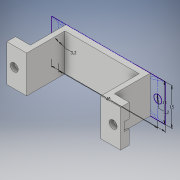
# Autodesk Inventor part: krepl_akum_line_racer
Saved by Autodesk Inventor 2019 (Build 230136000, 136)
## iProperties
Created: 2019-06-10
Part Number: krepl_akum_line_racer
Material: Типовые
Document SubType Name: Modeling
Designer: Администратор
Density: 1 g/cm^3
Appearance: По умолчанию
Author: Администратор
Autodesk Inventor part; units mm, degrees
ref_plane "YZ Plane" through (0, 0, 0) normal (1, 0, 0) x (0, 1, 0)
ref_plane "XZ Plane" through (0, 0, 0) normal (0, 1, 0) x (-1, 0, 0)
ref_plane "XY Plane" through (0, 0, 0) normal (0, 0, 1) x (1, 0, 0)
sketch "Эскиз1" plane through (0, 0, 0) normal (0, 0, 1) x (1, 0, 0)
  line L0 (-23, 7.5) -> (23, 7.5)
  line L1 (23, 7.5) -> (23, -7.5)
  line L2 (23, -7.5) -> (-23, -7.5)
  line L3 (-23, -7.5) -> (-23, 7.5)
  line L4 (-23, 7.5) -> (23, -7.5) construction
  line L5 (23, 7.5) -> (-23, -7.5) construction
  line L6 (-20, 7.5) -> (20, 7.5) construction
  line L7 (20, 7.5) -> (20, -7.5) construction
  line L8 (20, -7.5) -> (-20, -7.5) construction
  line L9 (-20, -7.5) -> (-20, 7.5) construction
  line L10 (-20, 7.5) -> (20, -7.5) construction
  line L11 (20, 7.5) -> (-20, -7.5) construction
  circle A0 centre (-20, 0) radius 1.6
  circle A1 centre (20, 0) radius 1.6
  point P0 (0, 0)
  dimension "d0" = 46
  dimension "d1" = 15
  dimension "d2" = 40
  dimension "d3" = 15
  dimension "d4" = 3.2
  dimension "d5" = 3.2
  constraints: 24 end point, 6 midpoint, 4 parallel, 2 centre point, 2 horizontal, 2 perpendicular
  measures "d0" distance of L1.end L2.end
  measures "d1" distance of L0.end L1.end
  measures "d2" distance of L7.end L8.end
  measures "d3" distance of L6.end L7.end
  measures "d4" diameter of A0
  measures "d5" diameter of A1
extrude "Выдавливание1" add sketch "Эскиз1" along normal blind 18
sketch "Эскиз2" plane through (0, 0, 18) normal (0, 0, 1) x (1, 0, 0)
  line L0 (-15, 7.5) -> (15, 7.5)
  line L1 (15, 7.5) -> (15, -7.5)
  line L2 (15, -7.5) -> (-15, -7.5)
  line L3 (-15, -7.5) -> (-15, 7.5)
  line L4 (-15, 7.5) -> (15, -7.5) construction
  line L5 (15, 7.5) -> (-15, -7.5) construction
  point P0 (0, 0)
  dimension "d8" = 30
  dimension "d9" = 15
  constraints: 12 end point, 2 midpoint, 2 parallel, 1 horizontal, 1 perpendicular
  measures "d8" distance of L1.end L2.end
  measures "d9" distance of L0.end L1.end
extrude "Выдавливание2" cut sketch "Эскиз2" against normal blind 15.5
sketch "Эскиз3" plane through (0, 0, 0) normal (0, 0, -1) x (-1, 0, 0)
  line L0 (-15, 7.5) -> (-15, -7.5) projected
  line L1 (15, -7.5) -> (15, 7.5) projected
  circle A0 centre (-20, 0) radius 1.6 projected
  circle A1 centre (20, 0) radius 1.6 projected
  line L2 (23, 7.5) -> (-23, 7.5) projected
  line L3 (-23, 7.5) -> (-23, -7.5) projected
  line L4 (-23, -7.5) -> (23, -7.5) projected
  line L5 (23, -7.5) -> (23, 7.5) projected
  line L6 (23, 7.5) -> (23, -7.5) projected
  line L7 (23, 7.5) -> (-23, 7.5) projected
  line L8 (23, -7.5) -> (17, -7.5)
  line L9 (17, -7.5) -> (17, 7.5)
  line L10 (17, 7.5) -> (23, 7.5)
  line L11 (23, 7.5) -> (23, -7.5)
  line L12 (-23, -7.5) -> (-23, 7.5) projected
  line L13 (-23, -7.5) -> (-17, -7.5)
  line L14 (-17, -7.5) -> (-17, 7.5)
  line L15 (-17, 7.5) -> (-23, 7.5)
  line L16 (-23, 7.5) -> (-23, -7.5)
  point P0 (0, 0)
  dimension "d18" = 6
  dimension "d20" = 6
  constraints: 16 end point, 4 parallel, 2 horizontal, 2 perpendicular, 2 point on line
  measures "d18" distance between parallel lines of L14 L3
  measures "d20" distance between parallel lines of L11 L9
extrude "Выдавливание3" cut sketch "Эскиз3" against normal blind 14.5 contours L14 L4 L3 L2 | L2 L5 L4 L9
sketch "Эскиз4" plane through (0, 0, 14.5) normal (0, 0, -1) x (-1, 0, 0)
  circle A0 centre (-20, 0) radius 1.6 projected
  line L0 (-17, -7.5) -> (-23, -7.5) projected
  line L1 (-23, 7.5) -> (-17, 7.5) projected
  line L2 (-23, -7.5) -> (-23, 7.5) projected
  circle A1 centre (20, 0) radius 1.6 projected
  line L3 (23, 7.5) -> (23, -7.5) projected
  line L4 (17, 7.5) -> (23, 7.5) projected
  line L5 (23, -7.5) -> (17, -7.5) projected
  line L6 (23, -1.7321) -> (20, -3.4641)
  line L7 (20, -3.4641) -> (17, -1.7321)
  line L8 (17, -1.7321) -> (17, 1.7321)
  line L9 (17, 1.7321) -> (20, 3.4641)
  line L10 (20, 3.4641) -> (23, 1.7321)
  line L11 (23, 1.7321) -> (23, -1.7321)
  line L12 (-23, 1.7321) -> (-20, 3.4641)
  line L13 (-20, 3.4641) -> (-17, 1.7321)
  line L14 (-17, 1.7321) -> (-17, -1.7321)
  line L15 (-17, -1.7321) -> (-20, -3.4641)
  line L16 (-20, -3.4641) -> (-23, -1.7321)
  line L17 (-23, -1.7321) -> (-23, 1.7321)
  line L18 (-17, -7.5) -> (-23, -7.5) projected
  line L19 (-23, 7.5) -> (-17, 7.5) projected
  line L20 (-23, -7.5) -> (-23, 7.5) projected
  line L21 (23, 7.5) -> (23, -7.5) projected
  line L22 (23, -7.5) -> (17, -7.5) projected
  line L23 (17, 7.5) -> (23, 7.5) projected
  line L24 (-17, 7.5) -> (-17, -7.5) projected
  line L25 (-17, 7.5) -> (-17, -7.5) projected
  line L26 (17, -7.5) -> (17, 7.5) projected
  line L27 (17, -7.5) -> (17, 7.5) projected
  point P0 (0, 0)
  dimension "d14" = 6
  dimension "d15" = 6
  constraints: 24 end point, 2 coincident, 26 other
  measures "d14" distance between parallel lines of L10 L7
  measures "d15" distance between parallel lines of L13 L16
extrude "Выдавливание4" cut sketch "Эскиз4" against normal blind 2 contours L15 L16 L2 L12 L13 L14 | L3 L6 L7 L8 L9 L10
